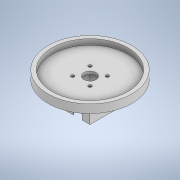
# Autodesk Inventor part: Основание
Saved by Autodesk Inventor 2021 (Build 250183000, 183)
## iProperties
Created: 2021-07-29
Part Number: Основание
Material: Типовые
Document SubType Name: Modeling
Designer: User
Density: 1 g/cm^3
Appearance: По умолчанию
Author: User
Autodesk Inventor part; units mm, degrees
ref_plane "YZ Plane" through (0, 0, 0) normal (1, 0, 0) x (0, 1, 0)
ref_plane "XZ Plane" through (0, 0, 0) normal (0, 1, 0) x (-1, 0, 0)
ref_plane "XY Plane" through (0, 0, 0) normal (0, 0, 1) x (1, 0, 0)
sketch "Эскиз1" plane through (0, 0, 0) normal (0, 1, 0) x (-1, 0, 0)
  circle A0 centre (0, 0) radius 75
  dimension "d0" = 150
  constraints: 1 centre point, 1 coincident
  measures "d0" diameter of A0
extrude "Выдавливание1" add sketch "Эскиз1" along normal blind 5
sketch "Эскиз2" plane through (0, 0, 0) normal (0, -1, 0) x (1, 0, 0)
  line L0 (21.175, 21.175) -> (-21.175, 21.175)
  line L1 (-21.175, 21.175) -> (-21.175, -21.175)
  line L2 (-21.175, -21.175) -> (21.175, -21.175)
  line L3 (21.175, -21.175) -> (21.175, 21.175)
  line L4 (21.175, 21.175) -> (-21.175, -21.175) construction
  line L5 (-21.175, 21.175) -> (21.175, -21.175) construction
  line L6 (22.175, 22.175) -> (-22.175, 22.175)
  line L7 (-22.175, 22.175) -> (-22.175, -22.175)
  line L8 (-22.175, -22.175) -> (22.175, -22.175)
  line L9 (22.175, -22.175) -> (22.175, 22.175)
  line L10 (22.175, 22.175) -> (-22.175, -22.175) construction
  line L11 (-22.175, 22.175) -> (22.175, -22.175) construction
  point P0 (0, 0)
  dimension "d3" = 42.35
  dimension "d4" = 42.35
  dimension "d5" = 44.35
  dimension "d6" = 44.35
  constraints: 24 end point, 4 midpoint, 4 parallel, 2 horizontal, 2 perpendicular
  measures "d3" distance of L2.end L1.end
  measures "d4" distance of L1.end L0.end
  measures "d5" distance of L8.end L7.end
  measures "d6" distance of L7.end L6.end
extrude "Выдавливание2" add sketch "Эскиз2" along normal blind 48
sketch "Эскиз4" plane through (-22.175, 0, 22.175) normal (0, 0, 1) x (1, 0, 0)
  line L0 (0, 0) -> (0, -48)
  line L1 (22.175, -48) -> (30.425, -48)
  line L2 (30.425, -48) -> (30.425, -38.5)
  line L3 (30.425, -38.5) -> (14.175, -38.5)
  line L4 (14.175, -38.5) -> (14.175, -48)
  line L5 (22.175, -48) -> (14.175, -48)
  point P0 (22.175, 0)
  dimension "d9" = 22.175
  dimension "d10" = 8.25
  dimension "d11" = 9.5
  dimension "d12" = 16.25
  constraints: 12 end point, 2 perpendicular, 1 vertical
  measures "d9" distance of L0.end L1.start
  measures "d10" distance of L1.start L1.end
  measures "d11" distance of L1.end L2.end
  measures "d12" distance of L2.end L3.end
extrude "Выдавливание3" cut sketch "Эскиз4" against normal blind 1
sketch "Эскиз5" plane through (0, 5, 0) normal (0, 1, 0) x (1, 0, 0)
  circle A0 centre (0, 0) radius 11
  line L0 (-15.5, -15.5) -> (15.5, -15.5)
  line L1 (15.5, -15.5) -> (15.5, 15.5)
  line L2 (15.5, 15.5) -> (-15.5, 15.5)
  line L3 (-15.5, 15.5) -> (-15.5, -15.5)
  line L4 (-15.5, -15.5) -> (15.5, 15.5) construction
  line L5 (15.5, -15.5) -> (-15.5, 15.5) construction
  circle A1 centre (15.5, 15.5) radius 2
  circle A2 centre (15.5, -15.5) radius 2
  circle A3 centre (-15.5, -15.5) radius 2
  circle A4 centre (-15.5, 15.5) radius 2
  dimension "d15" = 22
  dimension "d16" = 31
  dimension "d17" = 31
  dimension "d18" = 4
  dimension "d19" = 4
  dimension "d20" = 4
  dimension "d21" = 4
  constraints: 12 end point, 5 centre point, 5 coincident, 2 midpoint, 2 parallel, 1 horizontal, 1 perpendicular
  measures "d15" diameter of A0
  measures "d16" distance of L2.end L1.end
  measures "d17" distance of L1.end L0.end
  measures "d18" diameter of A1
  measures "d19" diameter of A2
  measures "d20" diameter of A3
  measures "d21" diameter of A4
extrude "Выдавливание4" cut sketch "Эскиз5" against normal blind 5 contours A0 | L3 A3 L0 | L0 A3 L3 | A2 L1 L0 | L0 L1 A2 | A4 L2 L3 | L3 L2 A4 | A1 L2 L1 | L1 L2 A1
sketch "Эскиз6" plane through (0, 5, 0) normal (0, 1, 0) x (1, 0, 0)
  circle A0 centre (15.5, 15.5) radius 2 projected
  line L0 (-15.5, -15.5) -> (15.5, -15.5)
  line L1 (15.5, -15.5) -> (15.5, 15.5)
  line L2 (15.5, 15.5) -> (-15.5, 15.5)
  line L3 (-15.5, 15.5) -> (-15.5, -15.5)
  line L4 (-15.5, -15.5) -> (15.5, 15.5) construction
  line L5 (15.5, -15.5) -> (-15.5, 15.5) construction
  circle A1 centre (15.5, 15.5) radius 3
  circle A2 centre (15.5, -15.5) radius 3
  circle A3 centre (-15.5, -15.5) radius 2 projected
  circle A4 centre (-15.5, -15.5) radius 3
  circle A5 centre (-15.5, 15.5) radius 2 projected
  circle A6 centre (-15.5, 15.5) radius 3
  point P0 (0, 0)
  dimension "d24" = 6
  dimension "d25" = 6
  dimension "d26" = 6
  dimension "d27" = 6
  constraints: 12 end point, 4 centre point, 4 coincident, 2 midpoint, 2 parallel, 1 horizontal, 1 perpendicular
  measures "d24" diameter of A1
  measures "d25" diameter of A2
  measures "d26" diameter of A4
  measures "d27" diameter of A6
extrude "Выдавливание5" cut sketch "Эскиз6" against normal blind 2 contours A0 L1 L2 | A0 L2 A1 L1 | L2 L1 A0 | A0 L1 A1 L2 | A6 L3 A5 L2 | L2 A5 L3 A6 | A2 L0 L1 | L1 L0 A2 | A5 L3 L2 | L2 L3 A5 | A4 L0 A3 L3 | L3 A3 L0 A4 | A3 L0 L3 | L3 L0 A3
sketch "Эскиз7" plane through (0, 5, 0) normal (0, 1, 0) x (1, 0, 0)
  circle A0 centre (0, 0) radius 67.9085
  circle A1 centre (0, 0) radius 75
  dimension "d30" = 135.817
  dimension "d31" = 150
  constraints: 2 centre point, 2 coincident
  measures "d30" diameter of A0
  measures "d31" diameter of A1
extrude "Выдавливание6" add sketch "Эскиз7" along normal blind 10
